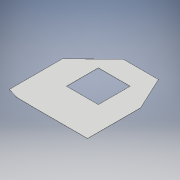
# Autodesk Inventor part: Cover V3.ipt-02
Saved by Autodesk Inventor 2018 (Build 220112000, 112)
## iProperties
Created: 2018-06-05
Part Number: Cover V3.ipt-02
Material: Generic
Document SubType Name: Modeling
Designer: P446509
Density: 1 g/cm^3
Appearance: Default
Author: P446509
Autodesk Inventor part; units mm, degrees
ref_plane "YZ Plane" through (0, 0, 0) normal (1, 0, 0) x (0, 1, 0)
ref_plane "XZ Plane" through (0, 0, 0) normal (0, 1, 0) x (-1, 0, 0)
ref_plane "XY Plane" through (0, 0, 0) normal (0, 0, 1) x (1, 0, 0)
ref_plane "Work Plane1" through (0, 0, 0) normal (0, 0, 1) x (1, 0, 0)
sketch "Sketch1" plane through (0, 0, 0) normal (0, 0, 1) x (1, 0, 0)
  line L0 (-429.9808, -407.4029) -> (-429.9808, -348.6109)
  line L1 (-324.2893, -437.4944) -> (-429.9808, -407.4029)
  line L2 (-219.5127, -437.4944) -> (-324.2893, -437.4944)
  line L3 (-219.5127, -439.0944) -> (-219.5127, -437.4944)
  line L4 (-429.9808, 92.5056) -> (-138.519, 375.9056)
  line L5 (-138.519, 375.9056) -> (191.481, 375.9056)
  line L6 (191.481, 375.9056) -> (338.3679, 60.9056)
  line L7 (338.3679, 60.9056) -> (338.3679, -439.0944)
  line L8 (338.3679, -439.0944) -> (-219.5127, -439.0944)
  line L9 (-429.9808, 92.5056) -> (-429.9808, -348.6109)
  circle A0 centre (-36.9222, 38.2477) radius 11.75
  line L10 (339.9679, -95.2638) -> (339.9679, -46.8324)
  circle A1 centre (-36.9222, 38.038) radius 60.05 construction
  circle A2 centre (-36.9222, 38.038) radius 65
  point P0 (0, 0)
extrude "Extrusion1" add sketch "Sketch1" along normal blind 1.6 contours L0 L9 L4 L5 L6 L7 L8 L3 L2 L1
sketch "Sketch2" plane through (0, 0, 1.6) normal (0, 0, 1) x (1, 0, 0)
  circle A0 centre (-36.9222, 38.038) radius 65 projected
  line L0 (-186.9222, -111.962) -> (113.0778, -111.962)
  line L1 (113.0778, -111.962) -> (113.0778, 188.038)
  line L2 (113.0778, 188.038) -> (-186.9222, 188.038)
  line L3 (-186.9222, 188.038) -> (-186.9222, -111.962)
  line L4 (-186.9222, -111.962) -> (113.0778, 188.038) construction
  line L5 (113.0778, -111.962) -> (-186.9222, 188.038) construction
  point P0 (0, 0)
  dimension "Door" = 300
  dimension "d25" = 300
  constraints: 12 end point, 2 midpoint, 2 parallel, 1 horizontal, 1 perpendicular
  measures "Door" distance of L2.end L1.end
  measures "d25" distance of L1.end L0.end
extrude "Extrusion2" cut sketch "Sketch2" against normal through all
sketch "Sketch3" plane through (0, 0, 1.6) normal (0, 0, 1) x (1, 0, 0)
  line L0 (-115.9127, -174.0672) -> (-113.9127, -174.0672) projected
  line L1 (-113.9127, -174.0672) -> (-113.9127, -304.5672) projected
  line L2 (-113.9127, -304.5672) -> (-115.9127, -304.5672) projected
  line L3 (-119.9127, -308.5672) -> (-115.9127, -304.5672) projected
  line L4 (-122.9127, -308.5672) -> (-119.9127, -308.5672) projected
  line L5 (-122.9127, -364.0672) -> (-122.9127, -308.5672) projected
  line L6 (-119.9127, -364.0672) -> (-122.9127, -364.0672) projected
  line L7 (-115.9127, -368.0672) -> (-119.9127, -364.0672) projected
  line L8 (-115.9127, -421.0944) -> (-115.9127, -368.0672) projected
  line L9 (-150.9127, -421.0944) -> (-115.9127, -421.0944) projected
  line L10 (-150.9127, -439.0944) -> (-150.9127, -421.0944) projected
  line L11 (87.7928, -439.0944) -> (-150.9127, -439.0944) projected
  line L12 (87.7928, -421.0944) -> (87.7928, -439.0944) projected
  line L13 (52.7928, -421.0944) -> (87.7928, -421.0944) projected
  line L14 (52.7928, -155.0944) -> (52.7928, -421.0944) projected
  arc A0 (56.7928, -151.0944) -> (52.7928, -155.0944) centre (56.7928, -155.0944) ccw projected
  line L15 (61.4116, -143.0944) -> (56.7928, -151.0944) projected
  line L16 (76.1116, -143.0944) -> (61.4116, -143.0944) projected
  line L17 (76.1116, -127.3944) -> (76.1116, -143.0944) projected
  line L18 (50.9116, -127.3944) -> (76.1116, -127.3944) projected
  line L19 (50.9116, -129.3944) -> (50.9116, -127.3944) projected
  line L20 (34.8116, -129.3944) -> (50.9116, -129.3944) projected
  line L21 (34.8116, -126.1944) -> (34.8116, -129.3944) projected
  line L22 (26.9979, -119.638) -> (34.8116, -126.1944) projected
  line L23 (23.1979, -119.638) -> (26.9979, -119.638) projected
  line L24 (15.0988, -129.2901) -> (23.1979, -119.638) projected
  line L25 (15.0988, -140.9901) -> (15.0988, -129.2901) projected
  line L26 (25.0988, -140.9901) -> (15.0988, -140.9901) projected
  line L27 (34.6251, -146.4901) -> (25.0988, -140.9901) projected
  spline S0 degree 4 poles (-91.6958, -146.9224) (-96.5362, -149.4958) (-101.3397, -154.9942) (-102.224, -165.1577) (-89.6958, -175.3075) (-29.4404, -181.638) (23.1944, -174.0672) (36.4189, -167.3497) (42.858, -156.2359) (37.7407, -148.2889) (34.6251, -146.4901) knots 0 0 0 0 0 1 2 3 4 5 6 7 7 7 7 7 projected
  line L28 (-87.6958, -139.9942) -> (-91.6958, -146.9224) projected
  line L29 (-77.0958, -139.9942) -> (-87.6958, -139.9942) projected
  line L30 (-75.5032, -127.3944) -> (-77.0958, -139.9942) projected
  line L31 (-111.7032, -127.3944) -> (-75.5032, -127.3944) projected
  line L32 (-111.7032, -129.3944) -> (-111.7032, -127.3944) projected
  line L33 (-130.7032, -129.3944) -> (-111.7032, -129.3944) projected
  line L34 (-130.7032, -127.3944) -> (-130.7032, -129.3944) projected
  line L35 (-139.188, -117.2826) -> (-130.7032, -127.3944) projected
  line L36 (-143.788, -117.2826) -> (-139.188, -117.2826) projected
  line L37 (-156.0447, -127.5672) -> (-143.788, -117.2826) projected
  line L38 (-156.0447, -141.5672) -> (-156.0447, -127.5672) projected
  line L39 (-142.0447, -141.5672) -> (-156.0447, -141.5672) projected
  line L40 (-140.3127, -144.5672) -> (-142.0447, -141.5672) projected
  line L41 (-122.9127, -144.5672) -> (-140.3127, -144.5672) projected
  line L42 (-122.9127, -167.0672) -> (-122.9127, -144.5672) projected
  arc A1 (-115.9127, -174.0672) -> (-122.9127, -167.0672) centre (-122.9127, -174.0672) ccw projected
  line L43 (-115.9127, -302.5672) -> (-115.9127, -176.0672)
  line L44 (-115.9127, -176.0672) -> (-118.3301, -176.0672)
  arc A2 (-118.3301, -176.0672) -> (-124.9127, -169.4846) centre (-122.9127, -174.0672) ccw
  line L45 (-124.9127, -169.4846) -> (-124.9127, -146.5672)
  line L46 (-124.9127, -146.5672) -> (-141.4674, -146.5672)
  line L47 (-141.4674, -146.5672) -> (-143.1994, -143.5672)
  line L48 (-143.1994, -143.5672) -> (-158.0447, -143.5672)
  line L49 (-158.0447, -143.5672) -> (-158.0447, -126.6346)
  line L50 (-158.0447, -126.6346) -> (-144.5159, -115.2826)
  line L51 (-144.5159, -115.2826) -> (-138.2554, -115.2826)
  line L52 (-138.2554, -115.2826) -> (-128.7032, -126.6665)
  line L53 (-128.7032, -126.6665) -> (-128.7032, -127.3944)
  line L54 (-128.7032, -127.3944) -> (-113.7032, -127.3944)
  line L55 (-113.7032, -127.3944) -> (-113.7032, -125.3944)
  line L56 (-113.7032, -125.3944) -> (-73.2345, -125.3944)
  line L57 (-73.2345, -125.3944) -> (-75.3327, -141.9942)
  line L58 (-75.3327, -141.9942) -> (-86.5411, -141.9942)
  line L59 (-86.5411, -141.9942) -> (-98.1431, -162.0894)
  line L60 (33.6251, -148.2222) -> (24.5629, -142.9901)
  line L61 (24.5629, -142.9901) -> (13.0988, -142.9901)
  line L62 (13.0988, -142.9901) -> (13.0988, -128.5622)
  line L63 (13.0988, -128.5622) -> (22.2653, -117.638)
  line L64 (22.2653, -117.638) -> (27.7259, -117.638)
  line L65 (27.7259, -117.638) -> (36.8116, -125.2618)
  line L66 (36.8116, -125.2618) -> (36.8116, -127.3944)
  line L67 (36.8116, -127.3944) -> (48.9116, -127.3944)
  line L68 (48.9116, -127.3944) -> (48.9116, -125.3944)
  line L69 (48.9116, -125.3944) -> (78.1116, -125.3944)
  line L70 (78.1116, -125.3944) -> (78.1116, -145.0944)
  line L71 (78.1116, -145.0944) -> (62.5663, -145.0944)
  line L72 (62.5663, -145.0944) -> (57.7928, -153.3624)
  arc A3 (57.7928, -153.3624) -> (54.7928, -155.0944) centre (56.7928, -155.0944) ccw
  line L73 (54.7928, -155.0944) -> (54.7928, -419.0944)
  line L74 (54.7928, -419.0944) -> (89.7928, -419.0944)
  line L75 (89.7928, -419.0944) -> (89.7928, -441.0944)
  line L76 (89.7928, -441.0944) -> (-152.9127, -441.0944)
  line L77 (-152.9127, -441.0944) -> (-152.9127, -419.0944)
  line L78 (-152.9127, -419.0944) -> (-117.9127, -419.0944)
  line L79 (-117.9127, -419.0944) -> (-117.9127, -368.8956)
  line L80 (-117.9127, -368.8956) -> (-120.7411, -366.0672)
  line L81 (-120.7411, -366.0672) -> (-124.9127, -366.0672)
  line L82 (-124.9127, -366.0672) -> (-124.9127, -306.5672)
  line L83 (-124.9127, -306.5672) -> (-120.7411, -306.5672)
  line L84 (-120.7411, -306.5672) -> (-116.7411, -302.5672)
  line L85 (-116.7411, -302.5672) -> (-115.9127, -302.5672)
  spline S1 degree 5 poles (-98.1431, -162.0894) (-97.9422, -162.7016) (-97.6824, -163.2943) (-97.3653, -163.8598) (-96.2561, -165.4674) (-94.7717, -166.7667) (-93.6914, -167.5033) (-90.5701, -169.2856) (-87.1826, -170.5186) (-85.001, -171.1946) (-79.4455, -172.6697) (-73.7957, -173.7283) (-70.3783, -174.2748) (-62.7102, -175.3204) (-55.0027, -176.0287) (-50.7343, -176.3328) (-42.0237, -176.7771) (-33.3024, -176.8728) (-28.8594, -176.8324) (-20.395, -176.5829) (-11.9473, -175.9969) (-7.9379, -175.6396) (-0.7832, -174.8598) (6.3364, -173.8114) (9.4652, -173.291) (14.7141, -172.3083) (19.9017, -171.0423) (21.9914, -170.4685) (25.4234, -169.3871) (28.7047, -167.9209) (29.9715, -167.2628) (32.144, -165.9026) (34.056, -164.2009) (34.8365, -163.3787) (36.1766, -161.6951) (37.1677, -159.7893) (37.5493, -158.8428) (38.0447, -156.8642) (37.9534, -154.8274) (37.7526, -153.8259) (37.0875, -151.8978) (35.954, -150.1975) (35.2802, -149.4242) (34.5075, -148.7324) (33.6251, -148.2222) knots 0 0 0 0 0 0 0.020543 0.020543 0.020543 0.062055 0.062055 0.062055 0.134898 0.134898 0.134898 0.245212 0.245212 0.245212 0.381631 0.381631 0.381631 0.523273 0.523273 0.523273 0.6516 0.6516 0.6516 0.752716 0.752716 0.752716 0.821812 0.821812 0.821812 0.867195 0.867195 0.867195 0.903189 0.903189 0.903189 0.935438 0.935438 0.935438 0.967522 0.967522 0.967522 1 1 1 1 1 1
  point P0 (0, 0)
  dimension "d28" = 2
  constraints: 86 end point, 4 point on circle, 2 centre point, 2 parallel, 46 other
  measures "d28" distance between parallel lines of L1 L43
extrude "Bed" [suppressed]
equation "\"d25\" = Door"
body "Solid1"
